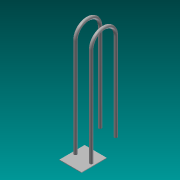
# Autodesk Inventor part: tangga naik
Saved by Autodesk Inventor 2014 SP2 (Build 180246200, 246)
## iProperties
Created: 2019-08-01
Part Number: tangga naik
Material: Steel, Mild
Document SubType Name: Modeling
Designer: USER PC
Density: 7.86 g/cm^3
Appearance: Steel
Author: USER PC
Autodesk Inventor part; units mm, degrees
sketch "Sketch1" plane through (0, 0, 0) normal (0, 0, 1) x (1, 0, 0)
  line L0 (0, 0) -> (350, 0)
  line L1 (350, 0) -> (350, -400)
  line L2 (350, -400) -> (0, -400)
  line L3 (0, -400) -> (0, 0)
  dimension "d0" = 350
  dimension "d1" = 400
  constraints: 8 end point, 2 parallel, 1 horizontal, 1 perpendicular
  measures "d0" distance of L1.end L2.end
  measures "d1" distance of L0.end L1.end
ref_plane "Work Plane1" through (0, 0, 50) normal (0, 0, 1) x (1, 0, 0)
extrude "Extrusion2" add sketch "Sketch1" along normal blind 10
sketch "Sketch3" plane through (0, 0, 10) normal (0, 0, 1) x (1, 0, 0)
  line L0 (350, 0) -> (0, 0) projected
  line L1 (0, 0) -> (0, -400) projected
  line L2 (350, -400) -> (350, 0) projected
  circle A0 centre (50, -195.4) radius 25.4
  circle A1 centre (50, -195.4) radius 19.9
  line L3 (175, 0) -> (175, -150)
  circle A2 centre (300, -195.4) radius 25.4
  circle A3 centre (300, -195.4) radius 19.9
  dimension "d11" = 50.8
  dimension "d12" = 5.5
  dimension "d13" = 150
  dimension "d15" = 50
  dimension "d16" = 195.4
  constraints: 4 centre point, 2 coincident, 2 end point, 2 symmetric about line, 1 midpoint, 1 parallel, 2 other
  measures "d11" diameter of A0
  measures "d12" radial gap between concentric circles of A0 A1
  measures "d13" distance of L3.start L3.end
  measures "d15" distance from line of A0.centre L1
  measures "d16" distance from line of A0.centre L0
extrude "Extrusion3" add sketch "Sketch3" along normal blind 1566
ref_plane "Work Plane2" through (0, 175.4, 0) normal (0, 1, 0) x (-1, 0, 0)
sketch "Sketch5" plane through (0, 0, 10) normal (0, 0, 1) x (1, 0, 0)
  circle A0 centre (50, -195.4) radius 25.4 projected
  circle A1 centre (300, -195.4) radius 25.4 projected
  line L0 (350, 0) -> (0, 0) projected
  line L1 (0, 0) -> (0, -400) projected
  line L2 (0, -400) -> (350, -400) projected
  line L3 (350, -400) -> (350, 0) projected
ref_plane "Work Plane3" through (0, 0, 1576) normal (0, 0, 1) x (1, 0, 0)
sketch "Sketch6" plane through (0, 0, 1576) normal (0, 0, 1) x (1, 0, 0)
  circle A0 centre (50, 195.4) radius 25.4
  circle A1 centre (50, 195.4) radius 19.9
  circle A2 centre (300, 195.4) radius 25.4
  circle A3 centre (300, 195.4) radius 19.9
  point P0 (0, 0)
  dimension "d25" = 50.8
  dimension "d26" = 5.5
  constraints: 4 centre point, 2 coincident
  measures "d25" diameter of A0
  measures "d26" radial gap between concentric circles of A0 A1
extrude "Extrusion4" add sketch "Sketch6" against normal blind 1400
sketch "Sketch8" plane through (0, 0, 0) normal (1, 0, 0) x (0, 1, 0)
  line L0 (0, 0) -> (0, 1576)
  line L1 (0, 1576) -> (0, 1796.8)
  dimension "d35" = 1576
  dimension "d36" = 220.8
  constraints: 4 end point, 1 coincident, 1 collinear, 1 vertical
  measures "d35" distance of L0.start L0.end
  measures "d36" distance of L0.end L1.end
sketch "Sketch9" plane through (0, 0, 0) normal (0, 1, 0) x (-1, 0, 0)
  line L0 (0, 1576) -> (0, 1796.8)
  circle A0 centre (-300, 1796.8) radius 25.4
  circle A1 centre (-300, 1796.8) radius 19.9
  point P0 (0, 0)
  dimension "d38" = 220.8
  dimension "d45" = 5.5
  constraints: 2 centre point, 2 coincident, 2 end point, 1 vertical
  measures "d38" distance of L0.start L0.end
  measures "d45" radial gap between concentric circles of A0 A1
sketch "Sketch10" plane through (300, 195.4, 1576) normal (0, 0, 1) x (1, 0, 0)
  circle A0 centre (0, 0) radius 19.9 projected
  circle A1 centre (0, 0) radius 25.4 projected
  circle A2 centre (0, 0) radius 25.4
  circle A3 centre (0, 0) radius 19.9
  point P0 (-300, -195.4)
  dimension "d47" = 50.8
  dimension "d48" = 5.5
  constraints: 2 centre point, 2 coincident
  measures "d47" diameter of A2
  measures "d48" radial gap between concentric circles of A2 A3
sketch "Sketch11" plane through (300, -195.4, 1576) normal (0, 0, 1) x (1, 0, 0)
  circle A0 centre (0, 0) radius 19.9 projected
  circle A1 centre (0, 0) radius 25.4 projected
  circle A2 centre (0, 0) radius 25.4
  circle A3 centre (0, 0) radius 19.9
  point P0 (-300, 195.4)
  dimension "d49" = 50.8
  dimension "d50" = 5.5
  constraints: 2 centre point, 1 coincident
  measures "d49" diameter of A2
  measures "d50" radial gap between concentric circles of A1 A3
sketch "Sketch12" plane through (50, 195.4, 1576) normal (0, 0, 1) x (1, 0, 0)
  circle A0 centre (0, 0) radius 19.9 projected
  circle A1 centre (0, 0) radius 25.4 projected
  circle A2 centre (0, 0) radius 25.4
  circle A3 centre (0, 0) radius 19.9
  point P0 (-50, -195.4)
  dimension "d51" = 50.8
  dimension "d52" = 5.5
  constraints: 2 centre point, 1 coincident
  measures "d51" diameter of A2
  measures "d52" radial gap between concentric circles of A1 A3
sketch "Sketch14" plane through (0, 0, 0) normal (0, 1, 0) x (-1, 0, 0)
  line L0 (0, 0) -> (0, 1576)
  line L1 (0, 1576) -> (0, 1796.8)
  circle A0 centre (-50, 1796.8) radius 25.4
  circle A1 centre (-50, 1796.8) radius 19.9
  dimension "d55" = 1576
  dimension "d56" = 220.8
  dimension "d58" = 50.8
  dimension "d59" = 5.5
  constraints: 4 end point, 2 centre point, 1 collinear, 1 vertical
  measures "d55" distance of L0.start L0.end
  measures "d56" distance of L0.end L1.end
  measures "d58" diameter of A0
  measures "d59" radial gap between concentric circles of A0 A1
sketch "Sketch15" plane through (50, -195.4, 1576) normal (0, 0, 1) x (1, 0, 0)
  circle A0 centre (0, 0) radius 19.9 projected
  circle A1 centre (0, 0) radius 25.4 projected
  circle A2 centre (0, 0) radius 25.4
  circle A3 centre (0, 0) radius 19.9
  point P0 (-50, 195.4)
  dimension "d60" = 50.8
  dimension "d61" = 5.5
  constraints: 2 centre point, 1 coincident
  measures "d60" diameter of A2
  measures "d61" radial gap between concentric circles of A1 A3
sketch "Sketch16" plane through (0, 0, 1576) normal (0, 0, 1) x (1, 0, 0)
  line L0 (0, 0) -> (50, 0)
  line L1 (50, 0) -> (50, 195.4)
  line L2 (50, 0) -> (50, -195.4)
  dimension "d62" = 50
  dimension "d63" = 195.4
  dimension "d64" = 195.4
  constraints: 6 end point, 1 collinear, 1 horizontal, 1 perpendicular
  measures "d62" distance of L0.start L0.end
  measures "d63" distance of L0.end L1.end
  measures "d64" distance of L0.end L2.end
ref_plane "Work Plane4" through (50, 0, 0) normal (1, 0, 0) x (0, 1, 0)
sketch "Sketch17" plane through (50, 0, 0) normal (1, 0, 0) x (0, 1, 0)
  line L0 (0, 0) -> (0, 1796.8)
  line L1 (0, 1796.8) -> (0, 1576)
  arc A0 (195.4, 1576) -> (-195.4, 1576) centre (0, 1576) ccw
  dimension "d66" = 1796.8
  dimension "d67" = 220.8
  dimension "d68" = 390.8
  constraints: 4 end point, 2 point on circle, 1 centre point, 1 coincident, 1 point on line, 1 vertical
  measures "d66" distance of L0.start L0.end
  measures "d67" distance of L0.end L1.end
  measures "d68" diameter of A0
sketch "Sketch18" plane through (300, 195.4, 1576) normal (0, 0, 1) x (1, 0, 0)
  circle A0 centre (0, 0) radius 19.9 projected
  circle A1 centre (0, 0) radius 25.4 projected
  point P0 (-300, -195.4)
sketch "Sketch19" plane through (300, -195.4, 1576) normal (0, 0, 1) x (1, 0, 0)
  circle A0 centre (0, 0) radius 19.9 projected
  circle A1 centre (0, 0) radius 25.4 projected
  line L0 (0, 0) -> (0, 195.4)
  line L1 (0, 0) -> (195.4, 0) construction
  line L2 (0, 195.4) -> (50, 195.4)
  point P0 (-300, 195.4)
  dimension "d69" = 195.4
  dimension "d70" = 90
  dimension "d71" = 50
  constraints: 6 end point, 2 perpendicular, 1 horizontal, 1 vertical
  measures "d69" distance of L0.start L0.end
  measures "d70" angle of L1 L0
  measures "d71" distance of L0.end L2.end
revolve "Revolution1" add sketch "Sketch19" angle 180 about axis through (300, 0, 1576) along (-1, 0, 0) contours A0 | A1
sketch "Sketch20" plane through (50, -195.4, 1576) normal (0, 0, 1) x (1, 0, 0)
  circle A0 centre (0, 0) radius 19.9 projected
  circle A1 centre (0, 0) radius 25.4 projected
  line L0 (0, 0) -> (0, 195.4)
  line L1 (0, 0) -> (195.4, 0) construction
  circle A2 centre (0, 0) radius 25.4
  line L2 (0, 195.4) -> (-50, 195.4)
  dimension "d73" = 195.4
  dimension "d74" = 90
  constraints: 6 end point, 1 centre point, 1 coincident, 1 concentric, 1 horizontal, 1 perpendicular, 1 vertical
  measures "d73" distance of L0.start L0.end
  measures "d74" angle of L1 L0
revolve "Revolution2" add sketch "Sketch20" angle 180 about axis through (50, 0, 1576) along (-1, 0, 0)
body "Solid2"
